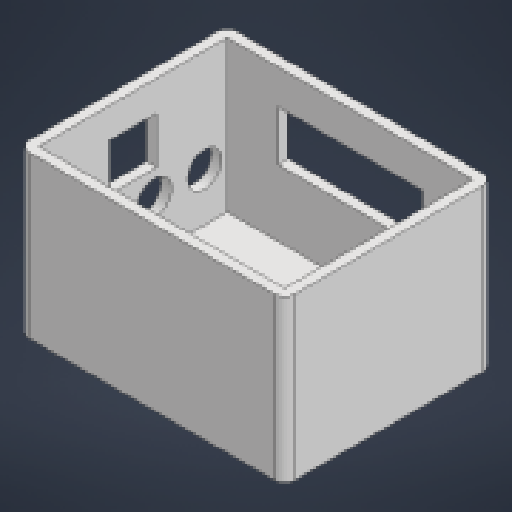
# Autodesk Inventor part: kucisteDonji
Saved by Autodesk Inventor 2025.2 (Build 292293000, 293)
## iProperties
Created: 2024-12-17
Part Number: kucisteDonji
Material: Generic
Document SubType Name: Modeling
Designer: antem
Density: 1 g/cm^3
Appearance: Default
Author: antem
Autodesk Inventor part; units mm, degrees
ref_plane "YZ Plane" through (0, 0, 0) normal (1, 0, 0) x (0, 1, 0)
ref_plane "XZ Plane" through (0, 0, 0) normal (0, 1, 0) x (-1, 0, 0)
ref_plane "XY Plane" through (0, 0, 0) normal (0, 0, 1) x (1, 0, 0)
sketch "Sketch1" plane through (0, 0, 0) normal (0, 1, 0) x (-1, 0, 0)
  line L0 (61, 46.75) -> (-61, 46.75)
  line L1 (-61, 46.75) -> (-61, -46.75)
  line L2 (-61, -46.75) -> (61, -46.75)
  line L3 (61, -46.75) -> (61, 46.75)
  line L4 (-61, 46.75) -> (61, -46.75) construction
  line L5 (66, 51.75) -> (-66, 51.75)
  line L6 (-66, 51.75) -> (-66, -51.75)
  line L7 (-66, -51.75) -> (66, -51.75)
  line L8 (66, -51.75) -> (66, 51.75)
  line L9 (0, -51.75) -> (0, -46.75) construction
  line L10 (66, 0) -> (61, 0) construction
  line L11 (58, 45.75) -> (1, 45.75) construction
  line L12 (1, 45.75) -> (1, -43.25) construction
  line L13 (1, -43.25) -> (58, -43.25) construction
  line L14 (58, -43.25) -> (58, 45.75) construction
  line L15 (-4, 35.25) -> (-60, 35.25) construction
  line L16 (-60, 35.25) -> (-60, -45.75) construction
  line L17 (-60, -45.75) -> (-4, -45.75) construction
  line L18 (-4, -45.75) -> (-4, 35.25) construction
  line L19 (1, 10) -> (-4, 10)
  line L20 (-4, 10) -> (-4, -10)
  line L21 (-4, -10) -> (1, -10)
  line L22 (1, -10) -> (1, 10)
  line L23 (1, -43.25) -> (-4, -43.25) construction
  line L24 (-1.5, -43.25) -> (-1.5, -10) construction
  line L25 (0, 0) -> (1, 0) construction
  dimension "d2" = 5
  dimension "d7" = 57
  dimension "d8" = 89
  dimension "d9" = 3.5
  dimension "d10" = 1
  dimension "d11" = 56
  dimension "d12" = 5
  dimension "d13" = 3
  dimension "d14" = 1
  dimension "d15" = 81
  dimension "d16" = 1
  dimension "d17" = 5
  dimension "d18" = 20
  constraints: 52 end point, 10 parallel, 8 midpoint, 7 horizontal, 7 perpendicular, 2 vertical, 1 coincident, 1 point on line
  measures "d2" distance between parallel lines of L6 L1
  measures "d7" distance of L12.end L13.end
  measures "d8" distance of L11.end L12.end
  measures "d9" distance between parallel lines of L2 L13
  measures "d10" distance between parallel lines of L11 L0
  measures "d11" distance of L16.end L17.end
  measures "d12" distance between parallel lines of L18 L12
  measures "d13" distance between parallel lines of L14 L3
  measures "d14" distance between parallel lines of L1 L16
  measures "d15" distance of L17.end L15.start
  measures "d16" distance between parallel lines of L2 L17
  measures "d17" distance between parallel lines of L22 L20
  measures "d18" distance between parallel lines of L21 L19
extrude "Extrusion1" add sketch "Sketch1" against normal blind 5 contours L3 L2 L1 L0 | L8 L7 L6 L5 | L22 L21 L20 L19
extrude "Extrusion2" add sketch "Sketch1" along normal blind 75 contours L8 L7 L6 L5
extrude "Extrusion3" add sketch "Sketch1" along normal blind 10 contours L22 L21 L20 L19
fillet "Fillet1" radius 5 4 edges at (66, 35, 51.75) (-66, 35, 51.75) (-66, 35, -51.75) (66, 35, -51.75)
sketch "Sketch2" plane through (-66, -5, -46.75) normal (-1, 0, 0) x (0, 0, 1)
  circle A0 centre (10.9794, 28.8313) radius 8.5 construction
  circle A1 centre (35.9794, 28.8313) radius 8.5 construction
  circle A2 centre (11.25, 29) radius 8.5
  circle A3 centre (36.25, 29) radius 8.5
  line L0 (10.9794, 28.8313) -> (35.9794, 28.8313) construction
  line L1 (11.25, 29) -> (36.25, 29) construction
  line L2 (93.5, 0) -> (0, 0) projected
  point P0 (46.75, 5)
  point P1 (23.75, 29)
  point P2 (46.75, 0)
  dimension "d26" = 29
  dimension "d27" = 23
  constraints: 4 end point, 2 centre point, 2 equal radius, 2 horizontal, 2 midpoint, 1 horizontal alignment, 1 parallel
  measures "d26" distance between parallel lines of L2 L1
  measures "d27" horizontal distance of point (46.75, 0) point (23.75, 29)
extrude "Extrusion4" cut sketch "Sketch2" against normal up to surface (5 mm away)
sketch "Sketch3" plane through (-66, -5, -46.75) normal (-1, 0, 0) x (0, 0, 1)
  line L0 (35.15, 65) -> (58.35, 65)
  line L1 (58.35, 65) -> (58.35, 41.8)
  line L2 (58.35, 41.8) -> (35.15, 41.8)
  line L3 (35.15, 41.8) -> (35.15, 65)
  line L4 (93.5, 0) -> (0, 0) projected
  line L5 (0, 80) -> (93.5, 80) projected
  point P0 (46.75, 5)
  point P1 (46.75, 0)
  point P2 (46.75, 41.8)
  dimension "d28" = 23.2
  dimension "d29" = 15
  constraints: 8 end point, 2 midpoint, 2 parallel, 2 perpendicular, 1 horizontal, 1 vertical alignment
  measures "d28" distance of L0.start L0.end
  measures "d29" distance between parallel lines of L5 L0
extrude "Extrusion5" cut sketch "Sketch3" against normal up to surface (5 mm away)
mirror "Mirror1" about plane through (0, 0, 0) normal (0, 0, 1) of "Extrusion4"
sketch "Sketch4" plane through (61, -5, -51.75) normal (0, 0, -1) x (-1, 0, 0)
  line L0 (25, 63) -> (97, 63)
  line L1 (97, 63) -> (97, 38)
  line L2 (97, 38) -> (25, 38)
  line L3 (25, 38) -> (25, 63)
  line L4 (0, 80) -> (122, 80) projected
  line L5 (24.8135, 37.7871) -> (96.8135, 37.7871) projected
  line L6 (96.8135, 37.7871) -> (96.8135, 62.7871) projected
  line L7 (96.8135, 62.7871) -> (24.8135, 62.7871) projected
  line L8 (24.8135, 62.7871) -> (24.8135, 37.7871) projected
  point P0 (61, 5)
  point P1 (61, 80)
  point P2 (61, 63)
  point P3 (25, 62.7871)
  point P4 (96.8135, 38)
  dimension "d32" = 72
  dimension "d33" = 25
  dimension "d34" = 17
  constraints: 8 end point, 2 midpoint, 2 parallel, 1 horizontal, 1 perpendicular, 1 vertical alignment
  measures "d32" distance of L0.start L0.end
  measures "d33" distance of L2.end L0.start
  measures "d34" distance between parallel lines of L4 L0
extrude "Extrusion6" cut sketch "Sketch4" against normal up to surface (5 mm away) contours L7 L6 L2 L3
body "Solid1"
